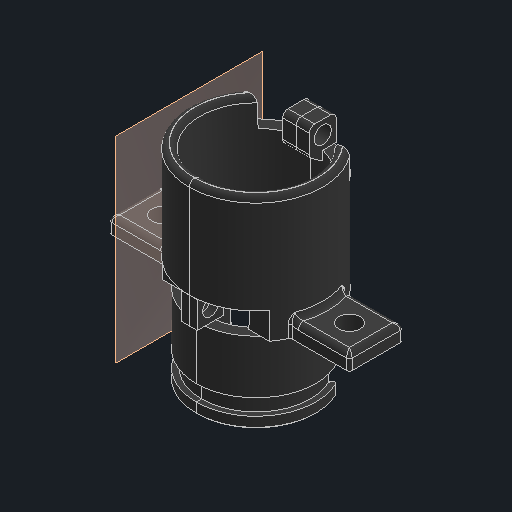
# Autodesk Inventor part: way
Saved by Autodesk Inventor 2026.1 (Build 301233020, 233B)
## iProperties
Created: 2025-12-16
Part Number: way
Material: 고무, 검은색
Document SubType Name: Modeling
Designer: jaewook
Density: 0.93 g/cm^3
Appearance: 고무 - 검은색
Author: jaewook
Autodesk Inventor part; units mm, degrees
ref_plane "XZ Plane" through (0, 0, 0) normal (0, 1, 0) x (-1, 0, 0)
ref_plane "XY Plane" through (0, 0, 0) normal (0, 0, 1) x (1, 0, 0)
sketch "스케치1" plane through (0, 0, 0) normal (0, 1, 0) x (-1, 0, 0)
  circle A0 centre (0, 0) radius 11.2
  circle A1 centre (0, 0) radius 9.2
  dimension "d0" = 2
  dimension "d1" = 22.4
  constraints: 2 centre point, 1 coincident
  measures "d0" radial gap between concentric circles of A0 A1
  measures "d1" diameter of A0
extrude "돌출1" add sketch "스케치1" along normal blind 15
sketch "스케치3" plane through (0, 0, 0) normal (1, 0, 0) x (0, 1, 0)
  line L0 (47.5, 0) -> (47.5, 12.5)
  line L1 (47.5, 12.5) -> (15, 12.5)
  line L2 (15, 12.5) -> (15, -17.7746)
  line L3 (15, -11.2) -> (15, 11.2) projected
  line L4 (0, -11.2) -> (0, 11.2) projected
  line L5 (47.5, 0) -> (15, 0)
  line L6 (15, 9.7) -> (38.5, 10.5)
  line L7 (38.5, 10.5) -> (38.5, 12.5)
  point P0 (0, 0)
  point P1 (0, 0)
  point P2 (15, 9.7)
  dimension "d7" = 0
  dimension "d8" = 12.5
  dimension "d9" = 32.5
  dimension "d10" = 1.5
  dimension "d11" = 2
  dimension "d12" = 9
  dimension "d21" = 23.5
  constraints: 12 end point, 4 perpendicular, 2 midpoint, 2 point on line, 1 collinear, 1 vertical
  measures "d7" vertical distance of point (0, 0) L5.end
  measures "d8" distance of L0.start L0.end
  measures "d9" distance between parallel lines of L2 L0
  measures "d10" distance of L3.end L6.start
  measures "d11" distance of L6.end L7.end
  measures "d12" distance between parallel lines of L7 L0
  measures "d21" distance between parallel lines of L2 L7
revolve "회전1" add sketch "스케치3" angle 360 about axis through (0, 47.5, 0) along (0, -1, 0) contours L7 L6 L2 L1
sketch "스케치5" plane through (0, 15, 0) normal (0, -1, 0) x (1, 0, 0)
  circle A0 centre (0, 0) radius 12.5 projected
  circle A1 centre (0, 0) radius 11.2 projected
  line L0 (0, 0) -> (0, 38.6929) construction
  line L1 (12.5, -5) -> (22.5, -5)
  line L2 (22.5, -5) -> (22.5, 5)
  line L3 (22.5, 5) -> (12.5, 5)
  line L4 (12.5, 5) -> (12.5, -5) construction
  line L5 (12.5, -5) -> (22.5, 5) construction
  line L6 (22.5, -5) -> (12.5, 5) construction
  line L7 (12.5, 5) -> (11.2492, 5)
  line L8 (11.2492, 5) -> (11.2492, -5)
  line L9 (11.2492, -5) -> (12.5, -5)
  circle A2 centre (17.5, 0) radius 2
  line L10 (-12.5, -5) -> (-22.5, -5)
  line L11 (-22.5, -5) -> (-22.5, 5)
  line L12 (-22.5, 5) -> (-12.5, 5)
  line L13 (-12.5, 5) -> (-12.5, -5) construction
  line L14 (-12.5, -5) -> (-22.5, 5) construction
  line L15 (-22.5, -5) -> (-12.5, 5) construction
  line L16 (-12.5, 5) -> (-11.2492, 5)
  line L17 (-11.2492, 5) -> (-11.2492, -5)
  line L18 (-11.2492, -5) -> (-12.5, -5)
  circle A3 centre (-17.5, 0) radius 2
  point P0 (11.4564, 5)
  point P1 (11.4564, -5)
  point P2 (-11.4564, -5)
  point P3 (-11.4564, 5)
  dimension "d16" = 10
  dimension "d17" = 10
  dimension "d18" = 4
  constraints: 38 end point, 8 symmetric about line, 3 perpendicular, 2 centre point, 2 coincident, 2 horizontal, 2 midpoint, 2 parallel, 1 horizontal alignment, 1 tangent, 1 vertical, 1 other
  measures "d16" distance of L1.end L2.end
  measures "d17" distance of L2.end L3.end
  measures "d18" diameter of A2
extrude "돌출4" add sketch "스케치5" against normal blind 3 contours A0 L7 L3 L2 L1 L9 | A0 L18 L10 L11 L12 L16
ref_plane "작업 평면1" through (-12.5, 26.75, 0) normal (1, 0, 0) x (0, 1, 0)
sketch "스케치6" plane through (-12.5, 26.75, 0) normal (1, 0, 0) x (0, 1, 0)
  line L0 (11.75, 12.5) -> (11.75, -12.5) projected
  line L1 (-11.75, 5) -> (-8.75, 5) projected
  line L2 (-8.75, 5) -> (-8.75, -5) projected
  line L3 (-8.75, -5) -> (-11.75, -5) projected
  line L4 (-11.75, -5) -> (-11.75, -5) projected
  line L5 (-11.75, -5) -> (-8.75, -5) projected
  line L6 (-8.75, -5) -> (-8.75, 5) projected
  line L7 (-8.75, 5) -> (-11.75, 5) projected
  line L8 (-11.75, 5) -> (-11.75, 5) projected
  line L9 (11.75, -12.5) -> (6.75, -12.5)
  line L10 (6.75, -12.5) -> (6.75, -7.5)
  line L11 (6.75, -7.5) -> (11.75, -7.5)
  line L12 (11.75, -7.5) -> (11.75, -12.5)
  point P0 (-26.75, 0)
  point P1 (11.75, -7.5)
  dimension "d22" = 5
  dimension "d23" = 5
  constraints: 8 end point, 2 parallel, 1 horizontal, 1 perpendicular
  measures "d22" distance of L10.end L11.end
  measures "d23" distance of L9.end L10.end
extrude "돌출5" cut sketch "스케치6" along normal blind 32
sketch "스케치7" plane through (0, 0, 0) normal (1, 0, 0) x (0, 1, 0)
  line L0 (33.5, -7.5) -> (33.5, -12.5) projected
  line L1 (38.5, -7.5) -> (33.5, -7.5) projected
  line L2 (33.5, -12.5) -> (38.5, -12.5)
  line L3 (38.5, -12.5) -> (38.5, -7.5)
  line L4 (38.5, -7.5) -> (33.5, -7.5)
  line L5 (33.5, -7.5) -> (33.5, -12.5)
  circle A0 centre (36, -10) radius 1.6
  line L6 (33.5, -7.5) -> (38.5, -7.5) projected
  line L7 (38.5, -7.5) -> (38.5, -7.5) projected
  line L8 (38.5, -7.5) -> (33.5, -7.5) projected
  line L9 (33.5, -7.5) -> (33.5, -7.5) projected
  line L10 (33.5, -7.5) -> (31.5586, -10.2637)
  line L11 (15, -9.7) -> (33.5, -10.3298) projected
  point P0 (0, 0)
  point P1 (15, 9.7)
  point P2 (15, -9.7)
  dimension "d26" = 3.2
  dimension "d27" = 2.5
  dimension "d28" = 2.5
  constraints: 10 end point, 2 parallel, 1 centre point, 1 horizontal, 1 perpendicular, 1 point on line
  measures "d26" diameter of A0
  measures "d27" distance from line of L2 A0.centre
  measures "d28" distance from line of L3 A0.centre
extrude "돌출6" add sketch "스케치7" along normal mid plane 5
fillet "모깎기1" radius 1 4 edges at (9.7211, 38.5, 3.9686) (-9.7211, 38.5, 3.9686) (-11.1803, 38.5, 5.5902) (11.1803, 38.5, 5.5902)
fillet "모깎기2" radius 1 8 edges at (-16.9782, 18, 5) (-22.5, 18, 0) (-16.9782, 18, -5) (-12.5, 18, 0) (16.9782, 18, 5) (12.5, 18, 0) (16.9782, 18, -5) (22.5, 18, 0)
fillet "모깎기3" radius 0.5 16 edges at (22.2071, 17.7071, 4.7071) (22.5, 16, 5) (22.2071, 17.7071, -4.7071) (22.5, 16, -5) (11.5366, 18.3613, 4.8121) (11.4564, 16.2791, 5) (11.5366, 18.3613, -4.8121) (11.4564, 16.2791, -5) (-11.5366, 18.3613, -4.8121) (-11.4564, 16.2791, -5) (-22.2071, 17.7071, -4.7071) (-22.5, 16, -5) (-22.2071, 17.7071, 4.7071) (-22.5, 16, 5) (-11.5366, 18.3613, 4.8121) (-11.4564, 16.2791, 5)
fillet "모깎기4" radius 0.5 1 edges at (9.2, 0, 0)
chamfer "모따기1" distance 0.2 angle 45 1 edges at (11.2, 0, 0)
fillet "모깎기5" radius 1 1 edges at (0, 33.5, -7.5)
fillet "모깎기6" radius 1 2 edges at (0, 38.5, -7.5) (0, 38.5, -12.5)
sketch "스케치8" plane through (0, 0, 0) normal (0, 0, 1) x (1, 0, 0)
  line L0 (-9.2, -5) -> (9.2, -5)
  line L1 (9.2, -5) -> (9.2, 5)
  line L2 (9.2, 5) -> (-9.2, 5)
  line L3 (-9.2, 5) -> (-9.2, -5)
  line L4 (-9.2, -5) -> (9.2, 5) construction
  line L5 (9.2, -5) -> (-9.2, 5) construction
  line L6 (11, 0) -> (-11, 0) projected
  point P0 (0, 0)
  point P1 (-9.2, 0)
  point P2 (9.2, 0)
  dimension "d40" = 5
  dimension "d41" = 18.4
  constraints: 12 end point, 2 midpoint, 2 parallel, 1 horizontal, 1 perpendicular
  measures "d40" distance between parallel lines of L6 L2
  measures "d41" distance of L1.end L2.end
extrude "돌출7" cut sketch "스케치8" against normal blind 15 contours L3 L2 L1 L6
sketch "스케치9" plane through (0, 0, 0) normal (0, 0, 1) x (1, 0, 0)
  line L0 (11.2, 0.2) -> (11.2, 15) projected
  line L1 (11.2, 5) -> (10.2, 5)
  line L2 (10.2, 5) -> (10.2, 2)
  line L3 (10.2, 2) -> (11.2, 2)
  line L4 (11.2, 2) -> (11.2, 5)
  line L5 (9.2, 5) -> (-9.2, 5) projected
  line L6 (0, 0) -> (0, 5)
  dimension "d44" = 1
  dimension "d45" = 3
  constraints: 10 end point, 2 parallel, 1 collinear, 1 horizontal, 1 midpoint, 1 perpendicular, 1 point on line
  measures "d44" distance of L1.start L1.end
  measures "d45" distance of L1.end L2.end
revolve "회전2" cut sketch "스케치9" angle 360 about axis through (0, 0, 0) along (0, 1, 0)
fillet "모깎기7" radius 1 1 edges at (0, 5, -9.2)
fillet "모깎기8" radius 0.5 2 edges at (-9.2, 1.1, -6.3875) (9.2, 1.1, -6.3875)
sketch "스케치10" plane through (0, 0, 0) normal (1, 0, 0) x (0, 1, 0)
  line L0 (37.5, 12.5) -> (15, 12.5) projected
  line L1 (15, 12.5) -> (20, 12.5)
  line L2 (20, 12.5) -> (20, 7.5)
  line L3 (20, 7.5) -> (15, 7.5)
  line L4 (15, 7.5) -> (15, 12.5)
  line L5 (15, 12.5) -> (15, 5.2885) projected
  point P0 (0, 0)
  dimension "d49" = 5
  dimension "d50" = 5
  constraints: 8 end point, 2 parallel, 1 collinear, 1 horizontal, 1 perpendicular, 1 point on line
  measures "d49" distance of L2.end L3.end
  measures "d50" distance of L1.end L2.end
extrude "돌출8" cut sketch "스케치10" along normal mid plane 30
sketch "스케치11" plane through (0, 0, 0) normal (1, 0, 0) x (0, 1, 0)
  line L0 (15, 7.5) -> (20, 7.5) projected
  line L1 (20, 7.5) -> (20, 12.5) projected
  line L2 (15, 7.5) -> (15, 11.2) projected
  line L3 (20, 7.5) -> (15, 7.5)
  line L4 (15, 7.5) -> (15, 12.5)
  line L5 (15, 12.5) -> (20, 12.5)
  line L6 (20, 12.5) -> (20, 7.5)
  circle A0 centre (17.5, 10) radius 1.5
  point P0 (0, 0)
  dimension "d53" = 5
  dimension "d54" = 5
  dimension "d55" = 3
  dimension "d56" = 2.5
  dimension "d57" = 2.5
  constraints: 8 end point, 2 parallel, 1 centre point, 1 horizontal, 1 perpendicular
  measures "d53" distance of L4.end L5.end
  measures "d54" distance of L3.end L4.end
  measures "d55" diameter of A0
  measures "d56" distance from line of L2 A0.centre
  measures "d57" distance from line of L5 A0.centre
extrude "돌출9" add sketch "스케치11" along normal mid plane 3
split body "분할1" result two bodies by plane through (0, 0, 0) normal (1, 0, 0) first body at (10.8435, 31.1788, 5.14)
